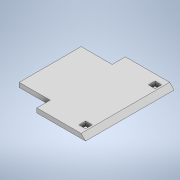
# Autodesk Inventor part: Helenowiak_podstawa
Saved by Autodesk Inventor 2021 (Build 250183000, 183)
## iProperties
Created: 2021-03-30
Part Number: Helenowiak_podstawa
Material: Ogólny
Document SubType Name: Modeling
Designer: jakub
Density: 1 g/cm^3
Appearance: Domyślna
Author: jakub
Autodesk Inventor part; units mm, degrees
ref_plane "YZ Plane" through (0, 0, 0) normal (1, 0, 0) x (0, 1, 0)
ref_plane "XZ Plane" through (0, 0, 0) normal (0, 1, 0) x (-1, 0, 0)
ref_plane "XY Plane" through (0, 0, 0) normal (0, 0, 1) x (1, 0, 0)
sketch "Szkic1" plane through (0, 0, 0) normal (0, 1, 0) x (-1, 0, 0)
  line L0 (0, 0) -> (-100, 0)
  line L1 (-100, 0) -> (-100, -100)
  line L2 (-100, -100) -> (0, -100)
  line L3 (0, -100) -> (0, 0)
  dimension "d0" = 100
  dimension "d1" = 100
  constraints: 8 end point, 2 parallel, 1 horizontal, 1 perpendicular
  measures "d0" distance of L2.end L1.end
  measures "d1" distance of L1.end L0.end
extrude "Wyciągnięcie proste1" add sketch "Szkic1" along normal blind 10
sketch "Szkic2" plane through (100, 0, -100) normal (0, 0, -1) x (-1, 0, 0)
  line L0 (0, 0) -> (5, 0)
  line L1 (5, 0) -> (15, 10)
  line L2 (0, 10) -> (100, 10) projected
  line L3 (5, 0) -> (19.1421, 0) construction
  line L4 (15, 10) -> (0, 10)
  line L5 (0, 10) -> (0, 0.5914)
  line L6 (0, 0) -> (100, 0) projected
  line L7 (0, 0.5914) -> (0, 0)
  line L8 (0, 0) -> (5, 0)
  dimension "d4" = 5
  dimension "d5" = 45
  constraints: 14 end point, 2 collinear, 2 horizontal, 2 perpendicular, 1 equal length, 1 point on line
  measures "d4" distance of L0.start L0.end
  measures "d5" angle of L3 L1
extrude "Wyciągnięcie proste2" cut sketch "Szkic2" against normal blind 100
sketch "Szkic4" plane through (0, 0, 0) normal (0, 0, 1) x (1, 0, 0)
  line L0 (0, 0) -> (100, 0)
  line L1 (100, 0) -> (100, 2)
  line L2 (100, 2) -> (0, 2)
  line L3 (0, 2) -> (0, 0)
  dimension "d8" = 100
  dimension "d9" = 2
  constraints: 8 end point, 2 parallel, 1 horizontal, 1 perpendicular
  measures "d8" distance of L2.end L1.end
  measures "d9" distance of L1.end L0.end
extrude "Wyciągnięcie proste3" cut sketch "Szkic4" against normal blind 100
sketch "Szkic5" plane through (0, 10, 0) normal (0, 1, 0) x (1, 0, 0)
  line L0 (0, 0) -> (85, 0) projected
  line L1 (0, 0) -> (35, 0)
  line L2 (35, 0) -> (35, 15)
  line L3 (35, 15) -> (0, 15)
  line L4 (0, 15) -> (0, 0)
  line L5 (0, 100) -> (0, 0) projected
  line L6 (0, 100) -> (35, 100)
  line L7 (35, 100) -> (35, 85)
  line L8 (35, 85) -> (0, 85)
  line L9 (0, 85) -> (0, 100)
  dimension "d12" = 35
  dimension "d13" = 15
  dimension "d14" = 35
  dimension "d15" = 15
  constraints: 16 end point, 4 parallel, 2 horizontal, 2 perpendicular
  measures "d12" distance of L3.end L2.end
  measures "d13" distance of L2.end L1.end
  measures "d14" distance of L7.end L8.end
  measures "d15" distance of L6.end L7.end
extrude "Wyciągnięcie proste4" cut sketch "Szkic5" against normal blind 100 contours L5 L6 L7 L8
sketch "Szkic6" plane through (0, 10, 0) normal (0, 1, 0) x (1, 0, 0)
  line L0 (0, 0) -> (93, 0) projected
  line L1 (0, 0) -> (35, 0)
  line L2 (35, 0) -> (35, 15)
  line L3 (35, 15) -> (0, 15)
  line L4 (0, 15) -> (0, 0)
  dimension "d18" = 35
  dimension "d19" = 15
  constraints: 8 end point, 2 parallel, 1 horizontal, 1 perpendicular
  measures "d18" distance of L3.end L2.end
  measures "d19" distance of L2.end L1.end
extrude "Wyciągnięcie proste5" cut sketch "Szkic6" against normal blind 100
sketch "Szkic7" plane through (35, 2, 0) normal (0, 0, 1) x (1, 0, 0)
  line L0 (58, 0) -> (50, 8) projected
  line L1 (58, 0) -> (-42, 0)
  line L2 (-42, 0) -> (-42, 2)
  line L3 (-42, 2) -> (58, 2)
  line L4 (58, 2) -> (58, 0)
  point P0 (-35, -2)
  point P1 (56, 2)
  dimension "d22" = 100
  dimension "d23" = 2
  constraints: 8 end point, 2 parallel, 1 horizontal, 1 perpendicular
  measures "d22" distance of L2.end L3.end
  measures "d23" distance of L1.end L2.end
extrude "Wyciągnięcie proste6" cut sketch "Szkic7" against normal blind 101.5 contours L1 L2 L3 L0
sketch "Szkic8" plane through (0, 10, 0) normal (0, 1, 0) x (1, 0, 0)
  line L0 (83, 93) -> (75.5, 93)
  line L1 (75.5, 93) -> (75.5, 85.5)
  line L2 (75.5, 85.5) -> (83, 85.5)
  line L3 (83, 85.5) -> (83, 93)
  point P0 (0, 0)
  dimension "d26" = 7.5
  dimension "d27" = 7.5
  constraints: 8 end point, 2 parallel, 1 horizontal, 1 perpendicular
  measures "d26" distance of L2.end L1.end
  measures "d27" distance of L1.end L0.end
extrude "Wyciągnięcie proste7" cut sketch "Szkic8" against normal blind 10
sketch "Szkic9" plane through (0, 10, 0) normal (0, 1, 0) x (1, 0, 0)
  line L0 (83, 7) -> (75.5, 7)
  line L1 (75.5, 7) -> (75.5, 14.5)
  line L2 (75.5, 14.5) -> (83, 14.5)
  line L3 (83, 14.5) -> (83, 7)
  point P0 (0, 0)
  dimension "d30" = 7.5
  dimension "d31" = 7.5
  constraints: 8 end point, 2 parallel, 1 horizontal, 1 perpendicular
  measures "d30" distance of L1.end L2.end
  measures "d31" distance of L0.end L1.end
extrude "Wyciągnięcie proste8" cut sketch "Szkic9" against normal blind 10
sketch "Szkic11" plane through (35, 10, 0) normal (0, 0, 1) x (1, 0, 0)
  line L0 (0, -6) -> (56, -6) projected
  line L1 (-35, 0) -> (-35, -6) projected
  line L2 (56, -6) -> (-35, -6)
  line L3 (-35, -6) -> (-35, -5)
  line L4 (-35, -5) -> (56, -5)
  line L5 (56, -5) -> (56, -6)
  point P0 (-35, -10)
  dimension "d34" = 1
  constraints: 8 end point, 2 parallel, 1 horizontal, 1 perpendicular, 1 point on line
  measures "d34" distance of L2.end L3.end
extrude "Wyciągnięcie proste9" cut sketch "Szkic11" against normal blind 100.75
